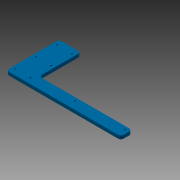
# Autodesk Inventor part: zCar_c
Saved by Autodesk Inventor 2013 (Build 170138000, 138)
## iProperties
Created: 2015-01-14
Part Number: zCar_c
Material: Generic
Document SubType Name: Modeling
Designer: dzban
Density: 1 g/cm^3
Author: dzban
Autodesk Inventor part; units mm, degrees
ref_plane "YZ Plane" through (0, 0, 0) normal (1, 0, 0) x (0, 1, 0)
ref_plane "XZ Plane" through (0, 0, 0) normal (0, 1, 0) x (-1, 0, 0)
ref_plane "XY Plane" through (0, 0, 0) normal (0, 0, 1) x (1, 0, 0)
sketch "Sketch1" plane through (0, 0, 0) normal (0, 0, 1) x (1, 0, 0)
  arc A0 (194.048, -0.1552) -> (189.048, 4.8448) centre (189.048, -0.1552) ccw
  line L0 (189.048, 4.8448) -> (32.048, 4.8448)
  arc A1 (27.048, 9.8448) -> (32.048, 4.8448) centre (32.048, 9.8448) ccw
  line L1 (27.048, 9.8448) -> (27.048, 74.8448)
  arc A2 (27.048, 74.8448) -> (22.048, 79.8448) centre (22.048, 74.8448) ccw
  line L2 (22.048, 79.8448) -> (-6.952, 79.8448)
  arc A3 (-6.952, 79.8448) -> (-11.952, 74.8448) centre (-6.952, 74.8448) ccw
  line L3 (-11.952, 74.8448) -> (-11.952, -10.1552)
  arc A4 (-11.952, -10.1552) -> (-6.952, -15.1552) centre (-6.952, -10.1552) ccw
  line L4 (-6.952, -15.1552) -> (189.048, -15.1552)
  arc A5 (189.048, -15.1552) -> (194.048, -10.1552) centre (189.048, -10.1552) ccw
  line L5 (194.048, -10.1552) -> (194.048, -0.1552)
  circle A6 centre (-6.252, 32.3448) radius 1.5
  circle A7 centre (21.348, 32.3448) radius 1.5
  circle A8 centre (-6.252, -5.1552) radius 1.5
  circle A9 centre (21.348, -5.1552) radius 1.5
  circle A10 centre (187.248, -1.3552) radius 1.5
  circle A11 centre (97.648, -1.3552) radius 1.5
  circle A12 centre (-6.252, 69.8448) radius 1.5
  circle A13 centre (21.348, 69.8448) radius 1.5
  point P0 (0, 0)
  point P1 (0, 0)
  constraints: 14 centre point, 12 end point, 12 point on circle
extrude "Extrusion1" add sketch "Sketch1" along normal blind 6
body "Solid1"
